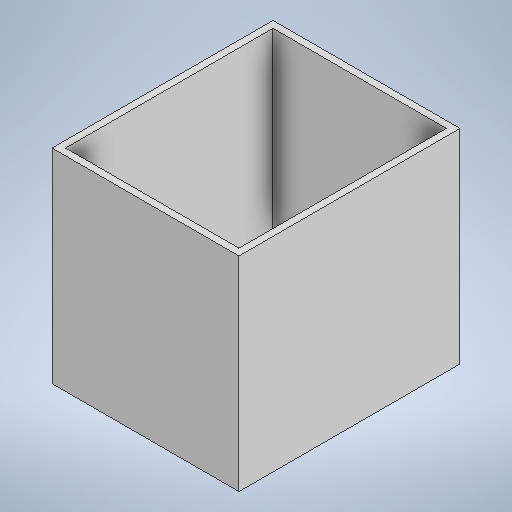
# Autodesk Inventor part: blankbox
Saved by Autodesk Inventor 2025 (Build 290162000, 162)
## iProperties
Created: 2024-07-25
Part Number: blankbox
Material: Generic
Document SubType Name: Modeling
Designer: ethan
Density: 1 g/cm^3
Appearance: Default
Author: ethan
Autodesk Inventor part; units mm, degrees
ref_plane "YZ Plane" through (0, 0, 0) normal (1, 0, 0) x (0, 1, 0)
ref_plane "XZ Plane" through (0, 0, 0) normal (0, 1, 0) x (-1, 0, 0)
ref_plane "XY Plane" through (0, 0, 0) normal (0, 0, 1) x (1, 0, 0)
sketch "Sketch1" plane through (0, 0, 0) normal (0, 1, 0) x (-1, 0, 0)
  line L0 (0, 0) -> (-64.77, 0)
  line L1 (0, 0) -> (0, -77.47)
  line L2 (0, 0) -> (-64.77, 0)
  line L3 (-64.77, 0) -> (-64.77, -77.47)
  line L4 (-64.77, -77.47) -> (0, -77.47)
  line L5 (0, -77.47) -> (0, 0)
  dimension "d0" = 64.77
  dimension "d1" = 77.47
  constraints: 12 end point, 2 horizontal, 2 parallel, 1 perpendicular, 1 vertical
  measures "d0" distance of L0.start L0.end
  measures "d1" distance of L0.start L1.end
extrude "Extrusion1" add sketch "Sketch1" along normal blind 2.54
sketch "Sketch2" plane through (0, 0, 0) normal (0, -1, 0) x (1, 0, 0)
  line L0 (0, -77.47) -> (0, 0) projected
  line L1 (64.77, -77.47) -> (0, -77.47) projected
  line L2 (64.77, 0) -> (64.77, -77.47) projected
  line L3 (0, 0) -> (64.77, 0) projected
  line L4 (67.31, 2.54) -> (67.31, -80.01)
  line L5 (67.31, -80.01) -> (-2.54, -80.01)
  line L6 (-2.54, -80.01) -> (-2.54, 2.54)
  line L7 (-2.54, 2.54) -> (67.31, 2.54)
  dimension "d4" = 2.54
  constraints: 8 end point, 3 other
  measures "d4" distance between parallel lines of L3 L7
extrude "Extrusion2" add sketch "Sketch2" against normal blind 76.2
body "Solid1"
